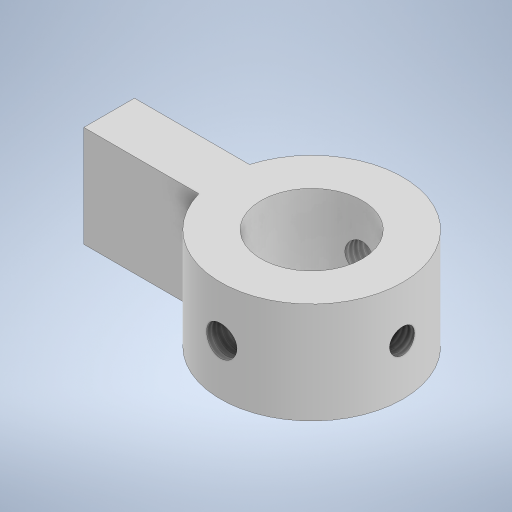
# Autodesk Inventor part: Стопор
Saved by Autodesk Inventor 2023 (Build 270158000, 158)
## iProperties
Created: 2022-04-28
Part Number: Стопор
Material: Типовые
Document SubType Name: Modeling
Designer: User
Density: 1 g/cm^3
Appearance: По умолчанию
Author: User
Autodesk Inventor part; units mm, degrees
ref_plane "YZ Plane" through (0, 0, 0) normal (1, 0, 0) x (0, 1, 0)
ref_plane "XZ Plane" through (0, 0, 0) normal (0, 1, 0) x (-1, 0, 0)
sketch "Эскиз1" plane through (0, 0, 0) normal (0, 1, 0) x (-1, 0, 0)
  circle A0 centre (0, 0) radius 5
  circle A1 centre (0, 0) radius 9
  line L0 (0, 0) -> (0, 2.5)
  line L1 (0, 2.5) -> (20, 2.5)
  line L2 (20, 2.5) -> (20, -2.5)
  line L3 (20, -2.5) -> (0, -2.5)
  point P0 (8.6458, 2.5)
  point P1 (8.6458, -2.5)
  dimension "d0" = 10
  dimension "d1" = 18
  dimension "d2" = 2.5
  dimension "d3" = 20
  dimension "d4" = 5
  constraints: 8 end point, 3 perpendicular, 2 centre point, 2 coincident, 1 point on line, 1 vertical
  measures "d0" diameter of A0
  measures "d1" diameter of A1
  measures "d2" distance of L0.start L0.end
  measures "d3" distance of L0.end L1.end
  measures "d4" distance of L1.end L2.end
extrude "Выдавливание1" add sketch "Эскиз1" along normal blind 10 contours A0 L1 A1 L3 | A0 L3 A1 L1 | L1 L2 L3 A1
sketch "Эскиз2" plane through (-20, 0, 2.5) normal (0, 0, 1) x (1, 0, 0)
  line L0 (0, 0) -> (0, 10) projected
  line L1 (0, 5) -> (20, 5)
  circle A0 centre (20, 5) radius 1.5
  point P0 (20, 0)
  dimension "d7" = 3
  constraints: 2 end point, 1 centre point, 1 coincident, 1 horizontal, 1 midpoint
  measures "d7" diameter of A0
extrude "Выдавливание2" cut sketch "Эскиз2" along normal mid plane 35.5
thread "Резьба1" size "M3x0.5" class "6H" standard "ISO Metric profile" full length
ref_plane "РабПлоскость1" through (10, 0, -2.5) normal (-1, 0, 0) x (0, 0, 1)
sketch "Эскиз3" plane through (0, 0, 0) normal (0, -1, 0) x (1, 0, 0)
  point P0 (0, 0)
sketch "Эскиз4" plane through (10, 0, -2.5) normal (-1, 0, 0) x (0, 0, 1)
  line L0 (2.5, 0) -> (2.5, 5)
  circle A0 centre (2.5, 5) radius 1.5
  dimension "d13" = 3
  constraints: 2 end point, 1 centre point, 1 coincident, 1 vertical
  measures "d13" diameter of A0
hole "Отверстие1" at (10, 5, 0) direction (-1, 0, 0) diameter 2.459 depth 8.8 thread size "M3x0.5" class "6H" standard "ISO Metric profile"
